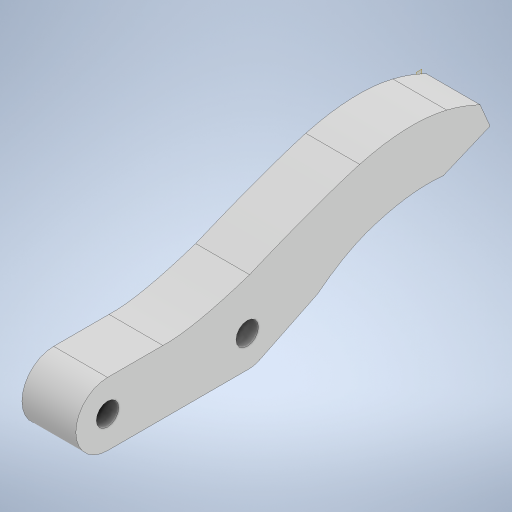
# Autodesk Inventor part: Final Gripper 1
Saved by Autodesk Inventor 2024.1 (Build 281209000, 209)
## iProperties
Created: 2023-12-01
Part Number: Final Gripper 1
Material: Generic
Document SubType Name: Modeling
Designer: vilas
Density: 1 g/cm^3
Appearance: Default
Author: vilas
Autodesk Inventor part; units mm, degrees
ref_plane "YZ Plane" through (0, 0, 0) normal (1, 0, 0) x (0, 1, 0)
ref_plane "XZ Plane" through (0, 0, 0) normal (0, 1, 0) x (-1, 0, 0)
ref_plane "XY Plane" through (0, 0, 0) normal (0, 0, 1) x (1, 0, 0)
ref_plane "Work Plane1" through (215.9, 467.0605, 68.1432) normal (1, 0, 0) x (0, 1, 0)
sketch "Sketch1" plane through (215.9, 467.0605, 68.1432) normal (1, 0, 0) x (0, 1, 0)
  line L0 (-213.126, 1464.2722) -> (-213.126, 1242.4656)
  spline S0 degree 2 poles (-213.126, 1242.4656) (-217.9428, 1125.9893) (-141.0804, 895.2277) knots 0 0 0 1 1 1
  spline S1 degree 2 poles (-141.0804, 895.2277) (-30.9453, 631.5803) (21.2303, 454.393) knots 0 0 0 1 1 1
  spline S2 degree 2 poles (21.2303, 454.393) (72.7957, 260.8739) (34.9413, 105.2911) knots 0 0 0 1 1 1
  spline S3 degree 2 poles (34.9413, 105.2911) (19.2909, 39.5013) (-13.3827, -28.1704) knots 0 0 0 1 1 1
  line L1 (-13.3827, -28.1704) -> (-107.2389, -68.1432)
  line L2 (-107.2389, -68.1432) -> (-185.683, 119.1347)
  spline S4 degree 2 poles (-185.683, 119.1347) (-171.2271, 262.5707) (-229.4608, 427.494) knots 0 0 0 1 1 1
  spline S5 degree 2 poles (-229.4608, 427.494) (-265.2584, 523.1386) (-344.3827, 623.2364) knots 0 0 0 1 1 1
  line L3 (-344.3827, 623.2364) -> (-467.0605, 875.6763)
  line L4 (-467.0605, 1464.2722) -> (-467.0605, 875.6763)
  arc A0 (-213.126, 1464.2722) -> (-467.0605, 1464.2722) centre (-340.0933, 1464.2722) ccw
  circle A1 centre (-340.0933, 1464.2722) radius 45
  circle A2 centre (-340.0933, 904.6692) radius 45
  point P0 (-467.0605, -68.1432)
  point P1 (-203.4806, 1128.5151)
  point P2 (-36.7776, 629.4713)
  point P3 (50.7616, 260.3303)
  point P4 (15.6727, 40.7996)
  point P5 (-188.3614, 260.3302)
  point P6 (-272.8905, 518.7472)
  dimension "d0" = 90
  dimension "d1" = 90
  dimension "d5" = 126.9673
  constraints: 10 end point, 3 centre point, 2 point on circle, 2 tangent, 2 vertical, 1 coincident, 18 other
  measures "d0" diameter of A1
  measures "d1" diameter of A2
  measures "d5" radius of A0
extrude "Extrusion1" add sketch "Sketch1" along normal blind 215.9
fillet "Fillet1" radius 100 1 edges at (323.85, 0, 943.8196)
body "Solid1"
